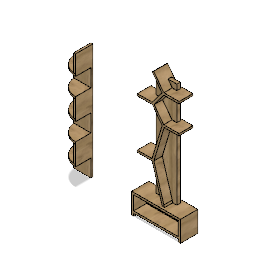
10-Day3 - Book Shelves v1 (Autodesk Fusion 360 design; units mm, degrees)
Autodesk Fusion 360 part; units mm, degrees
note: some values were not read from the file. Chosen so that the rebuilt part matches the saved one: a direction; which face or edge a step refers to.
sketch "Sketch1" plane through (0, 0, 0) normal (0, 0, 1) x (1, 0, 0)
  line L0 (700, 300) -> (0, 300)
  line L1 (0, 300) -> (0, 0)
  line L2 (700, 300) -> (700, 0)
  line L3 (670, 270) -> (670, 70)
  line L4 (30, 270) -> (30, 70)
  line L5 (670, 270) -> (30, 270)
  line L6 (30, 40) -> (670, 40)
  line L7 (30, 40) -> (30, 0)
  line L8 (670, 40) -> (670, 0)
  line L9 (0, 0) -> (30, 0)
  line L10 (670, 0) -> (700, 0)
  line L11 (30, 70) -> (670, 70)
  dimension "d2" = -30
  constraint horizontal L9
  constraint horizontal L0
  constraint vertical L1
  constraint coincident L1.end L9.start
  constraint perpendicular L3 L6
  constraint parallel L2 L3
  constraint parallel L1 L4
  constraint parallel L0 L5
  constraint perpendicular L7 L9
  constraint coincident L8.end L9
  constraint perpendicular L8 L9
  constraint collinear L9 L10
extrude "Extrude1" add sketch "Sketch1" along normal blind 200 and the other way blind 50 makes body 1
extrude "Extrude2" add sketch "Sketch1" along normal mid plane 30 contours L3 L4 L5 L11 bodies 1
sketch "Sketch2" plane through (0, 300, 0) normal (0, 1, 0) x (-1, 0, 0)
  line L0 (0, -50) -> (0, 200)
  line L1 (0, 200) -> (-700, 200)
  line L2 (-700, 200) -> (-700, -50)
  line L3 (-700, -50) -> (0, -50)
  line L4 (-200, 50) -> (-200, 0)
  line L5 (-200, 0) -> (-500, 0)
  line L6 (-500, 0) -> (-500, 50)
  line L7 (-500, 50) -> (-200, 50)
  constraint perpendicular L4 L5
  constraint perpendicular L5 L6
  constraint perpendicular L4 L7
extrude "Extrude3" add sketch "Sketch2" along normal blind 1500 contours L4 L5 L6 L7 bodies 1
sketch "Sketch4" plane through (0, 0, 50) normal (0, 0, 1) x (1, 0, 0)
  line L0 (200, 300) -> (500, 300)
  line L1 (500, 300) -> (500, 1800)
  line L2 (500, 1800) -> (200, 1800)
  line L3 (200, 1800) -> (200, 300)
  line L4 (433.0068, 330) -> (290.6605, 804.4878)
  line L5 (290.6605, 804.4878) -> (437.0432, 1292.4302)
  line L6 (430.2932, 1322.4302) -> (293.75, 1504.4878)
  line L7 (293.75, 1504.4878) -> (432.5, 1689.4878)
  line L8 (432.5, 1719.4878) -> (286.9996, 1913.4875)
  line L9 (440, 300) -> (410.6859, 300)
  line L10 (410.6859, 300) -> (263.8395, 789.4878)
  line L11 (263.8395, 819.4878) -> (408.4568, 1301.5454)
  line L12 (408.4568, 1301.5454) -> (267.5, 1489.4878)
  line L13 (267.5, 1519.4878) -> (406.25, 1704.4878)
  line L14 (406.25, 1704.4878) -> (262.9997, 1895.4875)
  line L15 (200, 789.4878) -> (263.8395, 789.4878)
  line L16 (200, 819.4878) -> (263.8395, 819.4878)
  line L17 (200, 819.4878) -> (200, 789.4878)
  line L18 (437.0432, 1292.4302) -> (500, 1292.4302)
  line L19 (430.2932, 1322.4302) -> (500, 1322.4302)
  line L20 (500, 1322.4302) -> (500, 1292.4302)
  line L21 (267.5, 1519.4878) -> (200, 1519.4878)
  line L22 (200, 1489.4878) -> (267.5, 1489.4878)
  line L23 (500, 1719.4878) -> (432.5, 1719.4878)
  line L24 (500, 1689.4878) -> (432.5, 1689.4878)
  line L25 (262.9997, 1895.4875) -> (286.9996, 1913.4875)
  line L26 (500, 1719.4878) -> (500, 1689.4878)
  line L27 (200, 1519.4878) -> (200, 1489.4878)
  line L28 (433.0068, 330) -> (440, 300)
  constraint horizontal L15
  constraint horizontal L16
  constraint perpendicular L15 L17
  constraint horizontal L18
  constraint horizontal L19
  constraint coincident L3 L21.end
  constraint perpendicular L3 L21
  constraint coincident L3 L22.start
  constraint perpendicular L3 L22
  constraint coincident L1 L23.start
  constraint coincident L1 L24.start
  constraint perpendicular L1 L24
  constraint perpendicular L8 L25
  constraint perpendicular L23 L26
  constraint collinear L0 L9
  constraint coincident L0 L9.start
extrude "Extrude4" add sketch "Sketch4" along normal blind 120 and the other way blind 80 separate body contours L0 L1 L2 L3 L4 L5 L6 L7 L8 L9 L10 L11 L12 L13 L14 L15 L16 L17 L18 L19 L20 L21 L22 L23 L24 L26 L27 L28 | L2 L8 L14 L25 makes body 2
extrude "Extrude5" add 2 faces at (500, 1312.4302, 103.3333) (500, 1709.4878, 103.3333) along direction (1, 0, 0) blind 120 separate body on bodies 2 makes body 3 at (540, 1322.4302, 36.6667) makes body 4 at (540, 1719.4878, 36.6667)
extrude "Extrude6" add 2 faces at (200, 1499.4878, 103.3333) (200, 799.4878, 103.3333) along direction (-1, 0, 0) blind 120 on bodies 2 bodies 2 1
combine "Combine1" operation add target body 2 tool bodies 4 3
extrude "Extrude7" add 2 faces at (620, 1709.4878, 103.3333) (620, 1312.4302, 103.3333) along direction (1, 0, 0) blind 30 on bodies 2 bodies 2
extrude "Extrude8" add 2 faces at (80, 1499.4878, 103.3333) (80, 799.4878, 103.3333) along direction (-1, 0, 0) blind 30 on bodies 2 bodies 2
move_body "Move1" bodies 2 to x (1, 0, 0) y (0, 1, 0) z (0, 0, 1) at (500, 0, 0)
sketch "Sketch5" plane through (0, 0, 0) normal (0, 0, 1) x (1, 0, 0)
  line L0 (0, 0) -> (-250, 0)
  line L1 (-250, 0) -> (-250, 250)
  line L2 (-250, 250) -> (0, 250)
  line L3 (0, 250) -> (0, 0)
  line L4 (-250, 250) -> (0, 250)
  line L5 (0, 250) -> (0, 280)
  line L6 (0, 280) -> (-250, 280)
  line L7 (-250, 280) -> (-250, 250)
  line L8 (0, 280) -> (-250, 280)
  line L9 (-250, 280) -> (-250, 530)
  line L10 (-250, 530) -> (0, 530)
  line L11 (0, 530) -> (0, 280)
  line L12 (-250, 530) -> (0, 530)
  line L13 (0, 530) -> (0, 560)
  line L14 (0, 560) -> (-250, 560)
  line L15 (-250, 560) -> (-250, 530)
  line L16 (0, 560) -> (-250, 560)
  line L17 (-250, 560) -> (-250, 810)
  line L18 (-250, 810) -> (0, 810)
  line L19 (0, 810) -> (0, 560)
  line L20 (-250, 810) -> (0, 810)
  line L21 (0, 810) -> (0, 840)
  line L22 (0, 840) -> (-250, 840)
  line L23 (-250, 840) -> (-250, 810)
  line L24 (0, 840) -> (-250, 840)
  line L25 (-250, 840) -> (-250, 1090)
  line L26 (-250, 1090) -> (0, 1090)
  line L27 (0, 1090) -> (0, 840)
  line L28 (-250, 1090) -> (0, 1090)
  line L29 (0, 1090) -> (0, 1120)
  line L30 (0, 1120) -> (-250, 1120)
  line L31 (-250, 1120) -> (-250, 1090)
  line L32 (0, 1120) -> (-250, 1120)
  line L33 (-250, 1120) -> (-250, 1370)
  line L34 (-250, 1370) -> (0, 1370)
  line L35 (0, 1370) -> (0, 1120)
  line L36 (-250, 1370) -> (0, 1370)
  line L37 (0, 1370) -> (0, 1400)
  line L38 (0, 1400) -> (-250, 1400)
  line L39 (-250, 1400) -> (-250, 1370)
  line L40 (0, 1400) -> (-250, 1400)
  line L41 (-250, 1400) -> (-250, 1650)
  line L42 (-250, 1650) -> (0, 1650)
  line L43 (0, 1650) -> (0, 1400)
  constraint horizontal L0
  constraint vertical L1
  constraint horizontal L2
  constraint vertical L3
  constraint coincident L0.start L3.end
  constraint horizontal L4
  constraint vertical L5
  constraint horizontal L6
  constraint vertical L7
  constraint horizontal L8
  constraint vertical L9
  constraint horizontal L10
  constraint vertical L11
  constraint horizontal L12
  constraint vertical L13
  constraint horizontal L14
  constraint vertical L15
  constraint horizontal L16
  constraint vertical L17
  constraint horizontal L18
  constraint vertical L19
  constraint horizontal L20
  constraint vertical L21
  constraint horizontal L22
  constraint vertical L23
  constraint horizontal L24
  constraint vertical L25
  constraint horizontal L26
  constraint vertical L27
  constraint horizontal L28
  constraint vertical L29
  constraint horizontal L30
  constraint vertical L31
  constraint horizontal L32
  constraint vertical L33
  constraint horizontal L34
  constraint vertical L35
  constraint horizontal L36
  constraint vertical L37
  constraint horizontal L38
  constraint vertical L39
  constraint horizontal L40
  constraint vertical L41
  constraint horizontal L42
  constraint vertical L43
ref_plane "WorkPlane1" through (-250, 0, 0) normal (1, 0, 0) x (0, 1, 0)
sketch "Sketch6" plane through (-250, 0, 0) normal (1, 0, 0) x (0, 0, -1)
  line L0 (0, 280) -> (250, 280)
  line L1 (250, 280) -> (250, 530)
  line L2 (250, 530) -> (0, 530)
  line L3 (0, 530) -> (0, 280)
  line L4 (0, 840) -> (250, 840)
  line L5 (250, 840) -> (250, 1090)
  line L6 (250, 1090) -> (0, 1090)
  line L7 (0, 1090) -> (0, 840)
  line L8 (0, 1400) -> (250, 1400)
  line L9 (250, 1400) -> (250, 1650)
  line L10 (250, 1650) -> (0, 1650)
  line L11 (0, 1650) -> (0, 1400)
  constraint horizontal L0
  constraint vertical L1
  constraint horizontal L2
  constraint vertical L3
  constraint perpendicular L1 L4
  constraint perpendicular L4 L5
  constraint perpendicular L5 L6
  constraint perpendicular L4 L7
  constraint perpendicular L5 L8
  constraint perpendicular L8 L9
  constraint perpendicular L9 L10
  constraint perpendicular L8 L11
delete_body "RemoveBody1" bodies 1
extrude "Extrude9" add sketch "Sketch5" against normal blind 30 separate body contours L0 L1 L2 L3 L4 | L14 L16 L17 L18 L19 L20 | L30 L32 L33 L34 L35 L36 makes body 5 at (-83.3333, 83.3333, 0) makes body 6 at (-83.3333, 643.3333, 0) makes body 7 at (-83.3333, 1203.3333, 0)
extrude "Extrude10" add sketch "Sketch6" along normal blind 30 separate body makes body 8 at (-250, 1566.6667, -83.3333) makes body 9 at (-250, 1006.6667, -83.3333) makes body 10 at (-250, 446.6667, -83.3333)
revolve "Revolve1" add sketch "Sketch5" angle 90 about axis through (-250, 560, 0) along (0, 1, 0) contours L2 L4 L5 L6 L7 L8 | L10 L12 L13 L14 L15 L16 | L18 L20 L21 L22 L23 L24 | L26 L28 L29 L30 L31 L32 | L34 L36 L37 L38 L39 L40 bodies 5 6 7 8 9 10
move_body "Move2" bodies 5 to x (-1, 0, 0) y (0, 1, 0) z (0, 0, -1) at (-500, 0, 0)
